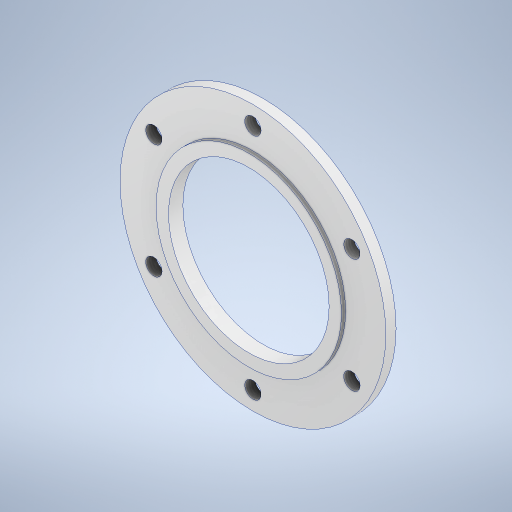
# Autodesk Inventor part: back
Saved by Autodesk Inventor 2023 (Build 270158000, 158)
## iProperties
Created: 2022-09-21
Part Number: back
Material: Aluminum 6061
Document SubType Name: Modeling
Designer: station
Density: 2.7 g/cm^3
Appearance: Aluminum - Flat
Author: station
Autodesk Inventor part; units mm, degrees
ref_plane "YZ Plane" through (0, 0, 0) normal (1, 0, 0) x (0, 1, 0)
ref_plane "XZ Plane" through (0, 0, 0) normal (0, 1, 0) x (-1, 0, 0)
ref_plane "XY Plane" through (0, 0, 0) normal (0, 0, 1) x (1, 0, 0)
sketch "Sketch1" plane through (0, 0, 0) normal (0, 0, 1) x (1, 0, 0)
  circle A0 centre (0, 0) radius 39
  circle A1 centre (0, 0) radius 42 construction
  circle A2 centre (0, 42) radius 3 construction
  circle A3 centre (0, 0) radius 37
  circle A4 centre (0, 0) radius 45
  circle A5 centre (0, 0) radius 64.5
  dimension "d5" = 84
  dimension "d0" = 78
  dimension "d6" = 6
  dimension "d14" = 74
  dimension "d15" = 90
  dimension "d16" = 129
  constraints: 5 centre point, 4 coincident, 1 vertical alignment, 2 other
  measures "d0" diameter of A0
  measures "d6" diameter of A2
  measures "d14" diameter of A3
  measures "d15" diameter of A4
  measures "d16" diameter of A5
extrude "Extrusion2" add sketch "Sketch1" along normal blind 5 contours A5
extrude "Extrusion3" add sketch "Sketch1" along normal blind 7 contours A4
sketch "Sketch2" plane through (0, 0, 0) normal (0, 0, -1) x (-1, 0, 0)
  circle A0 centre (0, 0) radius 55.5
  circle A1 centre (0, 55.5) radius 4
  dimension "d21" = 111
  dimension "d22" = 8
  constraints: 1 centre point, 1 coincident, 1 vertical alignment, 2 other
  measures "d22" diameter of A1
extrude "Extrusion4" cut sketch "Sketch2" against normal through all contours A1 A0 | A0 A1 picked at (-0.157, 54.1653) picked at (0.1387, 56.8154)
pattern_circular "Circular Pattern1" count 6 over 360 about axis through (0, 0, -10) along (0, 0, 1) of "Extrusion4"
thread "Thread1" size "M8x1.25" class "6H" standard "ANSI Metric M Profile" full length
thread "Thread2" size "M8x1.25" class "6H" standard "ANSI Metric M Profile" full length
thread "Thread3" size "M8x1.25" class "6H" standard "ANSI Metric M Profile" full length
thread "Thread4" size "M8x1.25" class "6H" standard "ANSI Metric M Profile" full length
thread "Thread5" size "M8x1.25" class "6H" standard "ANSI Metric M Profile" full length
thread "Thread6" size "M8x1.25" class "6H" standard "ANSI Metric M Profile" full length
body "Solid2"
